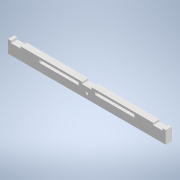
# Autodesk Inventor part: Lateral_Carril
Saved by Autodesk Inventor 2022 (Build 260153000, 153)
## iProperties
Created: 2022-01-30
Part Number: Lateral_Carril
Material: Generic
Document SubType Name: Modeling
Designer: katha
Density: 1 g/cm^3
Appearance: Default
Author: katha
Autodesk Inventor part; units mm, degrees
ref_plane "YZ Plane" through (0, 0, 0) normal (1, 0, 0) x (0, 1, 0)
ref_plane "XZ Plane" through (0, 0, 0) normal (0, 1, 0) x (-1, 0, 0)
ref_plane "XY Plane" through (0, 0, 0) normal (0, 0, 1) x (1, 0, 0)
sketch "Sketch1" plane through (0, 0, 0) normal (0, 0, 1) x (1, 0, 0)
  line L0 (125, -10) -> (-125, -10)
  line L1 (-125, -10) -> (-125, 10)
  line L2 (-125, 10) -> (125, 10)
  line L3 (125, 10) -> (125, -10)
  line L4 (125, -10) -> (-125, 10) construction
  line L5 (-125, -10) -> (125, 10) construction
  line L6 (75, 6.75) -> (-75, 6.75)
  line L7 (-75, 6.75) -> (-75, 2.25)
  line L8 (-75, 2.25) -> (75, 2.25)
  line L9 (75, 2.25) -> (75, 6.75)
  line L10 (75, 6.75) -> (-75, 2.25) construction
  line L11 (-75, 6.75) -> (75, 2.25) construction
  circle A0 centre (0, -2) radius 2
  line L12 (-13, 2.25) -> (-13, 6.75)
  line L13 (0, -2) -> (0, 4.5) construction
  line L14 (13, 2.25) -> (13, 6.75)
  line L15 (-120, 10) -> (-120, 6.8)
  line L16 (-120, 6.8) -> (-105, 6.8)
  line L17 (-105, 6.8) -> (-105, 10)
  line L18 (0, 10) -> (0, 6.8)
  line L19 (0, 6.8) -> (-7.5, 6.8)
  line L20 (-7.5, 6.8) -> (-7.5, 10)
  line L21 (-125, -10) -> (125, 10) construction
  line L22 (120, 10) -> (120, 6.8)
  line L23 (120, 6.8) -> (105, 6.8)
  line L24 (105, 6.8) -> (105, 10)
  line L25 (0, 6.8) -> (7.5, 6.8)
  line L26 (7.5, 6.8) -> (7.5, 10)
  point P0 (0, 0)
  point P1 (0, 4.5)
  point P2 (0, 0)
  point P3 (0, 0)
  dimension "d0" = 250
  dimension "d1" = 20
  dimension "d20" = 150
  dimension "d21" = 4.5
  dimension "d22" = 4.5
  dimension "d32" = 4
  dimension "d33" = 2
  dimension "d36" = 13
  dimension "d39" = 3.2
  dimension "d40" = 5
  dimension "d41" = 15
  dimension "d42" = 3.2
  dimension "d44" = 7.5
  constraints: 54 end point, 8 midpoint, 8 symmetric about line, 6 perpendicular, 6 point on line, 4 horizontal, 4 parallel, 2 vertical alignment, 1 centre point, 1 vertical
  measures "d0" distance of L1.end L2.end
  measures "d1" distance of L0.end L1.end
  measures "d20" distance of L8.end L7.end
  measures "d21" distance between parallel lines of L6 L8
  measures "d22" distance of point (0, 4.5) point (0, 0)
  measures "d32" diameter of A0
  measures "d33" distance of L13.start point (0, 0)
  measures "d36" distance from line of L12 point (0, 4.5)
  measures "d39" distance of L15.start L15.end
  measures "d40" distance between parallel lines of L1 L15
  measures "d41" distance of L15.end L16.end
  measures "d42" distance of L18.start L18.end
  measures "d44" distance of L18.end L19.end
extrude "Extrusion5" add sketch "Sketch1" along normal blind 3.2 contours L0 L1 L2 L15 L16 L17 L20 L19 L25 L26 L24 L23 L22 L3 | L14 L8 L12 L6
body "Solid4"
